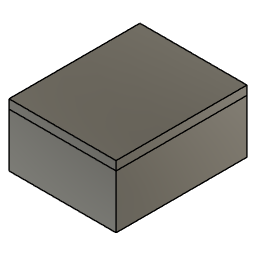
boxwlid v1 (Autodesk Fusion 360 design; units mm, degrees)
Autodesk Fusion 360 part; units mm, degrees
box "BoxPrimitive1" add length 220 width 180 height 90 placed x (0, 1, 0) y (-1, 0, 0) z (0, 0, 1) at (180, 0, 0) makes body 1
shell "Shell1" thickness 15 removed faces 1 at (120, 73.3333, 90) on bodies 1
sketch "Sketch2" plane through (0, 0, 90) normal (0, 0, 1) x (-1, 0, 0)
  line L0 (-165, -205) -> (-165, -15)
  line L1 (-165, -15) -> (-15, -15)
  line L2 (-15, -15) -> (-15, -205)
  line L3 (-15, -205) -> (-165, -205)
  line L4 (-180, -220) -> (0, -220)
  line L5 (0, -220) -> (0, 0)
  line L6 (0, 0) -> (-180, 0)
  line L7 (-180, 0) -> (-180, -220)
  line L8 (0, -220) -> (-180, -220)
  line L9 (-180, -220) -> (-180, 0)
  line L10 (-180, 0) -> (0, 0)
  line L11 (0, 0) -> (0, -220)
  constraint horizontal L8
  constraint vertical L9
  constraint horizontal L10
  constraint vertical L11
  constraint coincident L6.end L7.start
  constraint coincident L4.end L5.start
extrude "Extrude1" add sketch "Sketch2" along normal blind 15 separate body contours L0 L1 L2 L3 | L4 L5 L6 L7 L8 L9 L10 L11 makes body 2
